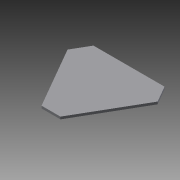
# Autodesk Inventor part: Frame Perimeter
Saved by Autodesk Inventor 2013 (Build 170138000, 138)
## iProperties
Created: 2013-01-21
Part Number: Frame Perimeter
Material: Generic
Document SubType Name: Modeling
Designer: carneeki
Density: 1 g/cm^3
Author: carneeki
Autodesk Inventor part; units mm, degrees
ref_plane "YZ Plane" through (0, 0, 0) normal (1, 0, 0) x (0, 1, 0)
ref_plane "XZ Plane" through (0, 0, 0) normal (0, 1, 0) x (-1, 0, 0)
ref_plane "XY Plane" through (0, 0, 0) normal (0, 0, 1) x (1, 0, 0)
sketch "Sketch1" plane through (0, 0, 0) normal (0, 1, 0) x (-1, 0, 0)
  line L0 (-219.7631, -36.0084) -> (-954.0508, -36.0084)
  line L1 (-954.0508, -36.0084) -> (-1055.6508, 139.968)
  line L2 (-1055.6508, 139.968) -> (-688.5069, 775.8798)
  line L3 (-688.5069, 775.8798) -> (-485.3069, 775.8798)
  line L4 (-485.3069, 775.8798) -> (-118.1631, 139.968)
  line L5 (-118.1631, 139.968) -> (-219.7631, -36.0084)
  line L6 (-586.9069, 775.8798) -> (-586.9069, 293.2798) construction
  line L7 (-1004.8508, 51.9798) -> (-586.9069, 293.2798) construction
  line L8 (-586.9069, 293.2798) -> (-168.9631, 51.9798) construction
  point P0 (0, 0)
  dimension "d8" = 203.2
  dimension "d9" = 120
  dimension "d10" = 120
  dimension "d13" = 203.2
  dimension "d17" = 203.2
  dimension "d21" = 482.6
  dimension "d22" = 120
  dimension "d23" = 120
  dimension "d24" = 482.6
  dimension "d25" = 482.6
  dimension "d26" = 734.2877
  dimension "d27" = 734.2877
  dimension "d28" = 734.2877
  constraints: 18 end point, 3 midpoint, 3 parallel, 2 perpendicular, 1 horizontal
  measures "d8" distance of L0.end L1.end
  measures "d9" angle of L0 L1
  measures "d10" angle of L1 L2
  measures "d13" distance of L2.end L3.end
  measures "d17" distance of L4.end L0.start
  measures "d21" distance of L6.start L6.end
  measures "d22" angle of L8 L6
  measures "d23" angle of L7 L6
  measures "d24" distance of L7.start L7.end
  measures "d25" distance of L7.end L8.end
  measures "d26" distance of L3.end L4.end
  measures "d27" distance of L1.end L2.end
  measures "d28" distance of L0.start L0.end
extrude "Extrusion1" add sketch "Sketch1" along normal blind 25.4
equation "\"d24\" = d21"
equation "\"d25\" = d21"
body "Solid1"
